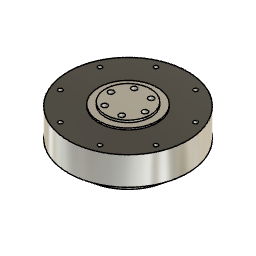
A80-6 motor body model (Autodesk Fusion 360 design; units mm, degrees)
description: Chassis model for making corresponding gear box
Autodesk Fusion 360 part; units mm, degrees
note: some values were not read from the file. Set by a fixed rule: which sketch regions a step uses.
sketch "Back plate disc" plane through (0, 0, 0) normal (0, 0, 1) x (1, 0, 0)
  circle A0 centre (0, 0) radius 49
  dimension "d21" = 98
  constraint coincident A0.centre origin
  measures "d21" diameter of A0
extrude "Main body extrude" add sketch "Back plate disc" along normal blind 23.2
sketch "Motor top outer ring sketch" plane through (0, 0, 23.2) normal (0, 0, 1) x (-1, 0, 0)
  circle A0 centre (0, 0) radius 49
  circle A1 centre (0, 0) radius 24
  dimension "d24" = 48
  constraint coincident A0.centre A1.centre
  measures "d24" diameter of A1
extrude "Motor top, outer ring extrude" add sketch "Motor top outer ring sketch" along normal blind 1.3 contours A1
sketch "Motor rotor ring sketch" plane through (0, 0, 24.5) normal (0, 0, 1) x (-1, 0, 0)
  circle A0 centre (0, 0) radius 24
  circle A1 centre (0, 0) radius 18.5
  dimension "d27" = 37
  constraint coincident A0.centre A1.centre
  measures "d27" diameter of A1
extrude "Motor rotor ring extrude" add sketch "Motor rotor ring sketch" along normal blind 1.7 contours A1
sketch "Motor driver cavity" plane through (0, 0, 0) normal (0, 0, 1) x (1, 0, 0)
  line L0 (-20.3145, 29.1131) -> (20.3145, 29.1131)
  arc A0 (-20.3145, 29.1131) -> (20.3145, 29.1131) centre (0, 0) ccw
  dimension "d30" = 71
  constraint coincident A0.centre origin
  constraint horizontal L0
  measures "d30" diameter of A0
extrude "Motor driver cavity extrude" add sketch "Motor driver cavity" against normal blind 11
sketch "Back plate mounting screws" plane through (0, 0, 0) normal (0, 0, -1) x (1, 0, 0)
  circle A0 centre (0, 0) radius 49
  circle A1 centre (0, 0) radius 42.5 construction
  circle A2 centre (16.1961, 39.293) radius 1.7
  circle A3 centre (-16.332, 39.2367) radius 1.7
  circle A4 centre (-39.293, 16.1961) radius 1.7
  circle A5 centre (-39.2367, -16.332) radius 1.7
  circle A6 centre (-16.1961, -39.293) radius 1.7
  circle A7 centre (16.332, -39.2367) radius 1.7
  circle A8 centre (39.293, -16.1961) radius 1.7
  circle A9 centre (39.2367, 16.332) radius 1.7
  line L0 (20.3145, -29.1131) -> (-20.3145, -29.1131)
  arc A10 (20.3145, -29.1131) -> (-20.3145, -29.1131) centre (0, 0) ccw
  dimension "d33" = 85
  dimension "d35" = 3.4
  dimension "d37" = 360
  measures "d33" diameter of A1
  measures "d35" diameter of A2
extrude "Representative M3 screw holes" cut sketch "Back plate mounting screws" against normal blind 2.5 contours A2 | A3 | A4 | A5 | A6 | A7 | A8 | A9
sketch "Top plate outer screw holes" plane through (0, 0, 23.2) normal (0, 0, 1) x (-1, 0, 0)
  circle A0 centre (0, 0) radius 24
  circle A1 centre (0, 0) radius 49
  circle A2 centre (0, 0) radius 42.5 construction
  circle A3 centre (-16.267, -39.2723) radius 1.7
  circle A4 centre (16.2672, -39.2722) radius 1.7
  circle A5 centre (39.2723, -16.267) radius 1.7
  circle A6 centre (39.2722, 16.2672) radius 1.7
  circle A7 centre (16.267, 39.2723) radius 1.7
  circle A8 centre (-16.2672, 39.2722) radius 1.7
  circle A9 centre (-39.2723, 16.267) radius 1.7
  circle A10 centre (-39.2722, -16.2672) radius 1.7
  dimension "d38" = 85
  dimension "d40" = 3.4
  dimension "d42" = 360
  constraint concentric A0 A2
  measures "d38" diameter of A2
  measures "d40" diameter of A3
extrude "Representative screw extrudes" cut sketch "Top plate outer screw holes" against normal blind 2.5 contours A3 | A4 | A5 | A6 | A7 | A8 | A9 | A10
sketch "Motor shaft screws" plane through (0, 0, 26.2) normal (0, 0, 1) x (-1, 0, 0)
  circle A0 centre (0, 0) radius 18.5
  circle A1 centre (0, 0) radius 14 construction
  circle A2 centre (-6.9901, -12.13) radius 2.2
  dimension "d56" = 28
  dimension "d58" = 4.4
  constraint concentric A0 A1
  measures "d56" diameter of A1
  measures "d58" diameter of A2
extrude "Motor shaft M4 screw extrude" cut sketch "Motor shaft screws" against normal blind 3.5 contours A2
pattern_circular "6 screws for rotor" count 6 over 360 about axis through (0, 0, 1.75) along (0, 0, 1) of "Motor shaft M4 screw extrude"
named bodies: "A80-6 motor body"
